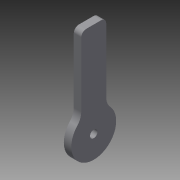
# Autodesk Inventor part: Camera Mount_A073113
Saved by Autodesk Inventor 2015 (Build 190159000, 159)
## iProperties
Created: 2013-05-28
Part Number: Camera Mount_A073113
Material: Generic
Document SubType Name: Modeling
Designer: Eric
Density: 1 g/cm^3
Appearance: Default
Author: Eric
Autodesk Inventor part; units mm, degrees
ref_plane "YZ Plane" through (0, 0, 0) normal (1, 0, 0) x (0, 1, 0)
ref_plane "XZ Plane" through (0, 0, 0) normal (0, 1, 0) x (-1, 0, 0)
ref_plane "XY Plane" through (0, 0, 0) normal (0, 0, 1) x (1, 0, 0)
sketch "Sketch1" plane through (0, 0, 0) normal (1, 0, 0) x (0, 1, 0)
  line L0 (-21, 41) -> (21, 41) construction
  line L1 (-5, 36) -> (-5, 10.198)
  line L2 (5, 36) -> (5, 10.198)
  arc A0 (-6.6, 6.1188) -> (6.6, 6.1188) centre (0, 0) ccw
  arc A1 (-6.6, 6.1188) -> (-5, 10.198) centre (-11, 10.198) ccw
  arc A2 (5, 10.198) -> (6.6, 6.1188) centre (11, 10.198) ccw
  arc A3 (-5, 45.7275) -> (5.2222, 45.7026) centre (0, 0) ccw construction
  circle A4 centre (0, 0) radius 1.5
  line L3 (-3, 38) -> (3, 38)
  arc A5 (-3, 38) -> (-5, 36) centre (-3, 36) ccw
  arc A6 (5, 36) -> (3, 38) centre (3, 36) ccw
  point P0 (-5, 38)
  point P1 (5, 38)
  point P2 (-5, 7.4833)
  point P3 (5, 7.4833)
  dimension "d25" = 10
  dimension "d69" = 6
  dimension "d101" = 3
  dimension "d108" = 9
  dimension "d109" = 38
  dimension "d110" = 5
  dimension "d111" = 2
  constraints: 14 point on circle, 8 end point, 8 tangent, 7 centre point, 6 point on line, 3 coincident, 2 equal radius, 1 parallel, 1 perpendicular, 1 vertical
  measures "d25" distance between parallel lines of L1 L2
  measures "d69" radius of A1
  measures "d101" diameter of A4
  measures "d108" radius of A0
  measures "d109" distance from line of L3 A0.centre
  measures "d110" distance from line of A0.centre L1
  measures "d111" radius of A5
extrude "Extrusion6" add sketch "Sketch1" along normal blind 3
body "Solid6"
